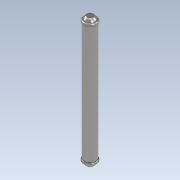
# Autodesk Inventor part: Eje-Bisagra
Saved by Autodesk Inventor 2021 (Build 250183000, 183)
## iProperties
Created: 2020-12-04
Part Number: Eje-Bisagra
Material: Acero inoxidable
Document SubType Name: Modeling
Designer: Yulitza
Density: 8 g/cm^3
Appearance: Semipulido
Author: Yulitza
Autodesk Inventor part; units mm, degrees
ref_plane "YZ Plane" through (0, 0, 0) normal (1, 0, 0) x (0, 1, 0)
ref_plane "XZ Plane" through (0, 0, 0) normal (0, 1, 0) x (-1, 0, 0)
ref_plane "XY Plane" through (0, 0, 0) normal (0, 0, 1) x (1, 0, 0)
sketch "Boceto1" plane through (0, 0, 0) normal (0, 1, 0) x (-1, 0, 0)
  circle A0 centre (0, 0) radius 4
  dimension "d0" = 8
  constraints: 1 centre point, 1 coincident
  measures "d0" diameter of A0
extrude "Extrusión1" add sketch "Boceto1" along normal mid plane 80
sketch "Boceto2" plane through (0, 0, 0) normal (1, 0, 0) x (0, 1, 0)
  line L0 (44, 0) -> (44, -2)
  line L1 (44, 0) -> (40, 0)
  line L2 (40, -4) -> (40, 4) projected
  line L3 (40, 0) -> (40, -3.6)
  arc A0 (40.0881, -4.0105) -> (41.9882, -3.753) centre (41, -3.6) ccw
  arc A1 (40, -4) -> (40.0881, -4.0105) centre (40.5168, -0.0335) ccw
  arc A2 (41.9882, -3.753) -> (44, -2) centre (40.5168, -0.0335) ccw
  point P0 (0, 0)
  dimension "d4" = 4
  dimension "d6" = 2
  dimension "d8" = 0.4
  constraints: 6 end point, 6 point on circle, 3 centre point, 1 collinear, 1 midpoint, 1 tangent, 1 vertical
  measures "d4" diameter of L0.end L1
  measures "d6" diameter of A0
  measures "d8" vertical distance of A0.centre L2.start
revolve "Revolución1" add sketch "Boceto2" angle 360 about axis through (0, 44, 0) along (0, -1, 0)
mirror "Simetría1" about plane through (0, 0, 0) normal (0, 1, 0) of "Revolución1"
